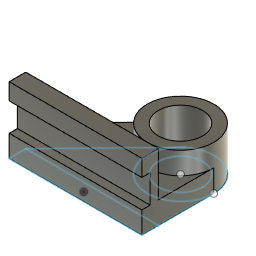
ex73 (Autodesk Fusion 360 design; units mm, degrees)
Autodesk Fusion 360 part; units mm, degrees
sketch "Sketch1" plane through (0, 0, 0) normal (0, 0, 1) x (1, 0, 0)
  line L0 (60, -7.5) -> (-60, -7.5)
  line L1 (-60, -7.5) -> (-60, 7.5)
  line L2 (-60, 7.5) -> (60, 7.5)
  line L3 (60, 7.5) -> (60, -7.5)
  line L4 (60, 7.5) -> (60, 57.5)
  circle A0 centre (30, 57.5) radius 30
  circle A1 centre (30, 57.5) radius 20
  line L5 (10.9888, 80.7072) -> (-60, 7.5)
  dimension "d1" = 120
  dimension "d2" = 15
  dimension "d5" = 30
  dimension "d6" = 60
  dimension "d7" = 40
  constraint horizontal L0
  constraint perpendicular L0 L1
  constraint parallel L0 L2
  constraint parallel L1 L3
  constraint perpendicular L2 L4
  constraint concentric A0 A1
  constraint coincident A0 L5.start
  measures "d1" distance of L1.end L2.end
  measures "d2" distance of L0.end L1.end
  measures "d5" distance of L4.end A0.centre
  measures "d6" diameter of A0
  measures "d7" diameter of A1
extrude "Extrude1" add sketch "Sketch1" along normal blind 40 contours A0 L5 picked at (10.8489, 75.8663)
extrude "Extrude2" add sketch "Sketch1" along normal blind 20 contours L2 L4 A0 L5
extrude "Extrude3" add sketch "Sketch1" along normal blind 60 contours L0 L1 L2 L3
sketch "Sketch2" plane through (-60, 0, 0) normal (-1, 0, 0) x (0, -1, 0)
  line L0 (-7.5, 0) -> (7.5, 0)
  line L1 (7.5, 0) -> (7.5, 60)
  line L2 (7.5, 60) -> (-7.5, 60)
  line L3 (-7.5, 60) -> (-7.5, 20)
  line L4 (-7.5, 20) -> (-7.5, 0)
  line L5 (7.5, 19.588) -> (0, 19.588)
  line L6 (0, 19.588) -> (0, 45)
  line L7 (0, 45) -> (7.5, 45)
  line L8 (7.5, 45) -> (7.5, 19.588)
  constraint horizontal L5
  constraint vertical L6
  constraint horizontal L7
  constraint vertical L8
  constraint coincident L1 L5.start
extrude "Extrude4" cut sketch "Sketch2" against normal blind 120 contours L1 L5 L6 L7 L8
